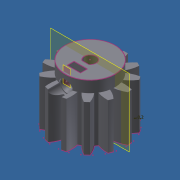
# Autodesk Inventor part: Stirnzahnrad2
Saved by Autodesk Inventor 2014 SP2 (Build 180246200, 246)
## iProperties
Created: 2014-12-12
Part Number: Stirnzahnrad2
Material: Steel
Document SubType Name: Modeling
Designer: 4ndreas
Categories: <?xml version="1.0" encoding="UTF-16"?> <MemberInstance><Categories><FamilyTemplate><FamilyTemplateParameter ValueType="xs:double" Id="1" ObjectReferenceKey="da_z" ObjectType="kUserParameterObject"/><FamilyTemplateParameter ValueType="xs:double" Id="2" ObjectReferenceKey="da_b" ObjectType="kUserParameterObject"/><FamilyTemplateParameter ValueType="xs:double" Id="3" ObjectReferenceKey="da_beta" ObjectType="kUserParameterObject"/><FamilyTemplateParameter ValueType="xs:double" Id="4" ObjectReferenceKey="da_da" ObjectType="kUserParameterObject"/><FamilyTemplateParameter ValueType="xs:double" Id="5" ObjectReferenceKey="da_aw" ObjectType="kUserParameterObject"/><FamilyTemplateParameter ValueType="xs:string" Id="6" ObjectReferenceKey="EAIAABAAAACIAQAAAAAAAIAAAAAAAAAA" ObjectType="83910656" SubObjectId="SurfaceGeometry"/></FamilyTemplate><ParamToTemplateMap><ParamToTemplate CategoryParameter="//CategoryParameter[@InternalName='046C89C9-8512-4d59-83FE-43B91F4F132A']" TemplateParameter="1"/><ParamToTemplate CategoryParameter="//CategoryParameter[@InternalName='2552DF32-E462-4b46-AEBF-C6C7768E72AC']" TemplateParameter="2"/><ParamToTemplate CategoryParameter="//CategoryParameter[@InternalName='C9EE641D-15FC-4fae-A226-E94C4372FDD7']" TemplateParameter="3"/><ParamToTemplate><ParamToTemplate CategoryParameter="//CategoryParameter[@InternalName='00B6519A-459B-49c7-AD84-2E56D39A5744']" ConstantValue="0.402671"/></ParamToTemplate><ParamToTemplate><ParamToTemplate CategoryParameter="//CategoryParameter[@InternalName='04B31F0E-C7A6-4894-AA32-9629BEFACF47']" ConstantValue="0.950000"/></ParamToTemplate><ParamToTemplate><ParamToTemplate CategoryParameter="//CategoryParameter[@InternalName='43CBEC2E-7847-49e7-A936-2F7889FCB2D9']" ConstantValue="0.500000"/></ParamToTemplate><ParamToTemplate><ParamToTemplate CategoryParameter="//CategoryParameter[@InternalName='B1EFC894-105D-4ebd-86BF-FA20ED196853']" ConstantValue="0.350000"/></ParamToTemplate><ParamToTemplate><ParamToTemplate CategoryParameter="//CategoryParameter[@InternalName='51175063-3D10-4879-93E8-6246FE8B403D']" ConstantValue="2060000000.000000"/></ParamToTemplate><ParamToTemplate><ParamToTemplate CategoryParameter="//CategoryParameter[@InternalName='A3A52E27-4454-46a9-B0BD-C932399B70AF']" ConstantValue="0.300000"/></ParamToTemplate><ParamToTemplate><ParamToTemplate CategoryParameter="//CategoryParameter[@InternalName='91B76062-C214-41d9-B1B9-14D2AB99603D']" ConstantValue="0.200000"/></ParamToTemplate><ParamToTemplate><ParamToTemplate CategoryParameter="//CategoryParameter[@InternalName='374E806E-8B8A-4dda-A9AA-1039D6500AD2']" ConstantValue="5.000000"/></ParamToTemplate><ParamToTemplate><ParamToTemplate CategoryParameter="//CategoryParameter[@InternalName='2D373A89-B862-43d6-8D0B-0CBF12AB9F6C']" ConstantValue="0.349066"/></ParamToTemplate><ParamToTemplate CategoryParameter="//CategoryParameter[@InternalName='37777632-D6A2-4fac-9D53-DB8ACD95C989']" TemplateParameter="4"/><ParamToTemplate CategoryParameter="//CategoryParameter[@InternalName='FD1017F1-B727-4f7e-9707-0F86F1FF9423']" TemplateParameter="5"/><ParamToTemplate><ParamToTemplate CategoryParameter="//CategoryParameter[@InternalName='9E1B4470-B2D3-4ff1-B813-535BB4CDF51A']" ConstantValue="3520000.000000"/></ParamToTemplate><ParamToTemplate><ParamToTemplate CategoryParameter="//CategoryParameter[@InternalName='F8452263-BFF6-458c-9FB1-07C4B99E95CD']" ConstantValue="11400000.000000"/></ParamToTemplate><ParamToTemplate><ParamToTemplate CategoryParameter="//CategoryParameter[@InternalName='3E3BB259-FD49-497f-8171-6EBC954A3479']" ConstantValue="2.000000"/></ParamToTemplate><ParamToTemplate CategoryParameter="//CategoryParameter[@InternalName='27C3BAF2-7550-4e4b-AE2C-0DB134B7D9B7']" TemplateParameter="6"/></ParamToTemplateMap><Category DisplayName="Gear" InternalName="DC85795E-93AB-48d5-8EEE-5A27447B64BD" Mnemonic="Gear"><CategoryParameter DisplayName="z" InternalName="046C89C9-8512-4d59-83FE-43B91F4F132A" Mnemonic="z"/><CategoryParameter DisplayName="b" InternalName="2552DF32-E462-4b46-AEBF-C6C7768E72AC" Mnemonic="b"/><CategoryParameter DisplayName="||b|" InternalName="C9EE641D-15FC-4fae-A226-E94C4372FDD7" Mnemonic="beta"/><CategoryParameter DisplayName="x" InternalName="00B6519A-459B-49c7-AD84-2E56D39A5744" Mnemonic="x"/><CategoryParameter DisplayName="a*" InternalName="04B31F0E-C7A6-4894-AA32-9629BEFACF47" Mnemonic="a"/><CategoryParameter DisplayName="c*" InternalName="43CBEC2E-7847-49e7-A936-2F7889FCB2D9" Mnemonic="c"/><CategoryParameter DisplayName="r|.f|*" InternalName="B1EFC894-105D-4ebd-86BF-FA20ED196853" Mnemonic="rf"/><CategoryParameter DisplayName="E" InternalName="51175063-3D10-4879-93E8-6246FE8B403D" Mnemonic="E"/><CategoryParameter DisplayName="||m|" InternalName="A3A52E27-4454-46a9-B0BD-C932399B70AF" Mnemonic="mi"/><Category DisplayName="SpurGear" InternalName="26C5A22E-A91E-4dfd-A3B3-23CCAFAE1764" Mnemonic="SpurGear"><CategoryParameter DisplayName="m" InternalName="91B76062-C214-41d9-B1B9-14D2AB99603D" Mnemonic="m"/><CategoryParameter DisplayName="P" InternalName="374E806E-8B8A-4dda-A9AA-1039D6500AD2" Mnemonic="PP"/><CategoryParameter DisplayName="||a|" InternalName="2D373A89-B862-43d6-8D0B-0CBF12AB9F6C" Mnemonic="alpha"/><CategoryParameter DisplayName="d|.a|" InternalName="37777632-D6A2-4fac-9D53-DB8ACD95C989" Mnemonic="da"/><CategoryParameter DisplayName="a|.w|" InternalName="FD1017F1-B727-4f7e-9707-0F86F1FF9423" Mnemonic="aw"/><CategoryParameter DisplayName="||s||.Flim|" InternalName="9E1B4470-B2D3-4ff1-B813-535BB4CDF51A" Mnemonic="sFlim"/><CategoryParameter DisplayName="||s||.Hlim|" InternalName="F8452263-BFF6-458c-9FB1-07C4B99E95CD" Mnemonic="sHlim"/><CategoryParameter DisplayName="Typ" InternalName="3E3BB259-FD49-497f-8171-6EBC954A3479" Mnemonic="type"/><CategoryParameter DisplayName="PitchDiameter" InternalName="27C3BAF2-7550-4e4b-AE2C-0DB134B7D9B7" Mnemonic="IDS_PITCHDIAM"/></Category></Category></Categories></MemberInstance>
Density: 1 g/cm^3
Appearance: Steel
CustomPartVersion: 1
Author: 4ndreas
Autodesk Inventor part; units mm, degrees
sketch "Sketch1" plane through (0, 0, 0) normal (0, 0, 1) x (1, 0, 0)
  circle A0 centre (0, 0) radius 15.6768
  dimension "d0" = 31.3535
  constraints: 1 centre point
  measures "d0" diameter of A0
extrude "Extrusion1" add sketch "Sketch1" along normal blind 20
ref_plane "Work Plane2" through (0, 0, 10) normal (0, 0, 1) x (1, 0, 0)
sketch "Sketch2" plane through (0, 0, 0) normal (0, 0, -1) x (-1, 0, 0)
  circle A0 centre (0, 0) radius 15.6768 projected
  circle A1 centre (0, 0) radius 13.1311
  dimension "d3" = 26.2623
  constraints: 1 centre point, 1 coincident
  measures "d3" diameter of A1
surface extrude "Flankendurchmesser" sketch "Sketch2" against normal through all shown no curves A1
ref_plane "Work Plane8" through (0, 0, 0) normal (0.9709418, 0.2393157, 0) x (0, 0, 1)
ref_plane "Work Plane9" through (0, 0, 0) normal (1, 0, 0) x (0, 1, 0)
spur gear teeth "Stirnzahnrad" teeth 13 pitch diameter 26 tip diameter 31.3535 root diameter 21.8107 face width 20 start plane through (0, 0, 0) normal (0, 0, -1) x (-1, 0, 0)
sketch "Skizze3" plane through (0, 0, 20) normal (0, 0, 1) x (1, 0, 0)
  arc A0 (-6.7255, 8.5845) -> (-7.7112, 7.7112) centre (0, 0) ccw projected
  arc A1 (-6.4339, 14.2956) -> (-8.1102, 13.4159) centre (0, 0) ccw projected
  circle A2 centre (0, 0) radius 10.9053
  constraints: 1 centre point, 1 coincident, 1 concentric
extrude "Extrusion2" add sketch "Skizze3" along normal blind 7
sketch "Skizze4" plane through (0, 0, 27) normal (0, 0, 1) x (1, 0, 0)
  circle A0 centre (0, 0) radius 10.9053 projected
  line L0 (-10.9053, 0) -> (10.9053, 0)
  constraints: 2 end point, 2 point on circle, 1 horizontal, 1 midpoint
ref_plane "Arbeitsebene11" through (-10.9053, 0, 27) normal (0, -1, 0) x (1, 0, 0)
hole "Bohrung1" at (0, 0, 27) direction (0, 0, -1) diameter 5.2 end through all
sketch "Skizze6" plane through (0, 0, 27) normal (0, 0, 1) x (1, 0, 0)
  circle A0 centre (0, 0) radius 2.6 projected
  circle A1 centre (0, 0) radius 10.9053 projected
  line L0 (-1.4913, -2.1298) -> (1.4913, -2.1298)
  line L1 (-1.4913, -2.1298) -> (-4.533, 0) construction
  line L2 (-4.533, 0) -> (0, 0) construction
  dimension "d63" = 35
  constraints: 6 end point, 2 point on circle, 1 horizontal, 1 parallel, 1 tangent
  measures "d63" angle of L1 L2
extrude "Extrusion4" add sketch "Skizze6" against normal up to surface (27 mm away) contours L0 A0 picked at (0.3106, -2.229)
sketch "Skizze5" plane through (-10.9053, 0, 27) normal (0, -1, 0) x (1, 0, 0)
  line L0 (10.2469, -27) -> (11.5638, -27) projected
  line L1 (-2.6508, -7) -> (0, -7) projected
  line L2 (0, -7) -> (0, 0) projected
  line L3 (13.5053, 0) -> (21.8107, 0) projected
  line L4 (21.8107, 0) -> (21.8107, -7) projected
  line L5 (21.8107, -7) -> (24.4615, -7) projected
  line L6 (24.4615, -7) -> (24.4615, -27) projected
  line L7 (24.4615, -27) -> (13.5053, -27) projected
  line L8 (-2.6508, -27) -> (-2.6508, -7) projected
  line L9 (0, -7) -> (21.8107, -7)
  circle A0 centre (10.9053, -7) radius 1.6
  line L10 (13.5053, -27) -> (13.5053, 0) projected
  line L11 (0, 0) -> (8.3053, 0) projected
  line L12 (8.3053, 0) -> (8.3053, -27) projected
  line L13 (8.3053, -27) -> (-2.6508, -27) projected
  point P0 (10.9053, -27)
  dimension "d52" = 3.2
  constraints: 2 end point, 1 centre point, 1 midpoint, 1 perpendicular
  measures "d52" diameter of A0
extrude "Extrusion3" cut sketch "Skizze5" along normal through all contours A0 L9 | L9 A0
sketch "Skizze7" plane through (0, 0, 27) normal (0, 0, 1) x (1, 0, 0)
  line L0 (1.4913, -2.1298) -> (-1.4913, -2.1298) projected
  circle A0 centre (0, 0) radius 10.9053 projected
  line L1 (-2.9, -4.1298) -> (2.9, -4.1298)
  line L2 (2.9, -4.1298) -> (2.9, -7.1298)
  line L3 (2.9, -7.1298) -> (-2.9, -7.1298)
  line L4 (-2.9, -7.1298) -> (-2.9, -4.1298)
  line L5 (0, 0) -> (0, -10.9053) construction
  dimension "d66" = 3
  dimension "d67" = 5.8
  dimension "d68" = 2
  constraints: 10 end point, 3 parallel, 1 horizontal, 1 perpendicular, 1 vertical alignment, 2 other
  measures "d66" distance between parallel lines of L3 L1
  measures "d67" distance between parallel lines of L2 L4
  measures "d68" distance between parallel lines of L1 L0
extrude "Extrusion5" cut sketch "Skizze7" against normal blind 12 contours L1 L2 L3 L4
ref_plane "Arbeitsebene12" through (-1.4913, -10.1298, 27) normal (0, 1, 0) x (1, 0, 0)
sketch "Skizze8" plane through (-1.4913, -10.1298, 27) normal (0, 1, 0) x (1, 0, 0)
  circle A0 centre (1.4913, 7) radius 1.6 projected
  line L0 (-2.5477, 0) -> (-2.5477, 7) projected
  line L1 (-2.5477, 7) -> (-3.0246, 7) projected
  line L2 (-3.0246, 7) -> (-3.0246, 27) projected
  line L3 (-3.0246, 27) -> (6.0072, 27) projected
  line L4 (6.0072, 27) -> (6.0072, 7) projected
  line L5 (6.0072, 7) -> (5.5303, 7) projected
  line L6 (5.5303, 7) -> (5.5303, 0) projected
  line L7 (5.5303, 0) -> (-2.5477, 0) projected
  line L8 (12.2006, 7) -> (7.9327, 7) projected
  line L9 (7.9327, 7) -> (7.9327, 27) projected
  line L10 (7.9327, 27) -> (12.2006, 27) projected
  line L11 (12.2006, 27) -> (12.2006, 7) projected
  line L12 (-4.9502, 7) -> (-9.218, 7) projected
  line L13 (-9.218, 7) -> (-9.218, 27) projected
  line L14 (-9.218, 27) -> (-4.9502, 27) projected
  line L15 (-4.9502, 27) -> (-4.9502, 7) projected
  circle A1 centre (1.4913, 7) radius 3
  point P0 (1.4913, 27)
  dimension "d72" = 6
  constraints: 1 centre point, 1 coincident
  measures "d72" diameter of A1
extrude "Extrusion6" cut sketch "Skizze8" against normal blind 12 contours A1
chamfer "Fase1" distance 1 angle 45 1 edges at (-1.6, -10.1298, 20)
sketch "Skizze10" plane through (0, 0, 27) normal (0, 0, 1) x (1, 0, 0)
  line L0 (-2.9, -7.1298) -> (-2.9, -4.1298) projected
  line L1 (-2.9, -4.1298) -> (2.9, -4.1298) projected
  line L2 (2.9, -4.1298) -> (2.9, -7.1298) projected
  line L3 (2.9, -7.1298) -> (-2.9, -7.1298) projected
  arc A0 (1.4913, -2.1298) -> (-1.4913, -2.1298) centre (0, 0) ccw projected
  line L4 (1.4913, -2.1298) -> (-1.4913, -2.1298) projected
  circle A1 centre (0, 0) radius 10.9053 projected
extrude "Extrusion7" cut sketch "Skizze10" against normal blind 2
sketch "Skizze11" plane through (0, 0, 0) normal (0, 0, -1) x (-1, 0, 0)
  arc A0 (1.4913, -2.1298) -> (-1.4913, -2.1298) centre (0, 0) ccw projected
  line L0 (-1.4913, -2.1298) -> (1.4913, -2.1298) projected
  arc A1 (6.7255, 8.5845) -> (8.1102, 13.4159) centre (-5.623, 14.7376) ccw projected
  arc A2 (8.1102, 13.4159) -> (6.4339, 14.2956) centre (0, 0) ccw projected
  arc A3 (6.4339, 14.2956) -> (3.2444, 10.4116) centre (15.323, 3.7443) ccw projected
  arc A4 (3.2444, 10.4116) -> (1.9657, 10.7267) centre (0, 0) ccw projected
  arc A5 (1.9657, 10.7267) -> (0.9465, 15.6482) centre (-11.8278, 10.4364) ccw projected
  arc A6 (0.9465, 15.6482) -> (-0.9465, 15.6482) centre (0, 0) ccw projected
  arc A7 (-0.9465, 15.6482) -> (-1.9657, 10.7267) centre (11.8278, 10.4364) ccw projected
  arc A8 (-1.9657, 10.7267) -> (-3.2444, 10.4116) centre (0, 0) ccw projected
  arc A9 (-3.2444, 10.4116) -> (-6.4339, 14.2956) centre (-15.323, 3.7443) ccw projected
  arc A10 (-6.4339, 14.2956) -> (-8.1102, 13.4159) centre (0, 0) ccw projected
  arc A11 (-8.1102, 13.4159) -> (-6.7255, 8.5845) centre (5.623, 14.7376) ccw projected
  arc A12 (-6.7255, 8.5845) -> (-7.7112, 7.7112) centre (0, 0) ccw projected
  arc A13 (-7.7112, 7.7112) -> (-12.3405, 9.6682) centre (-15.308, -3.8056) ccw projected
  arc A14 (-12.3405, 9.6682) -> (-13.4159, 8.1102) centre (0, 0) ccw projected
  arc A15 (-13.4159, 8.1102) -> (-9.9446, 4.4757) centre (-1.87, 15.6627) ccw projected
  arc A16 (-9.9446, 4.4757) -> (-10.4116, 3.2444) centre (0, 0) ccw projected
  arc A17 (-10.4116, 3.2444) -> (-15.42, 2.8258) centre (-11.786, -10.4836) ccw projected
  arc A18 (-15.42, 2.8258) -> (-15.6482, 0.9465) centre (0, 0) ccw projected
  arc A19 (-15.6482, 0.9465) -> (-10.8854, -0.6584) centre (-8.9346, 12.9995) ccw projected
  arc A20 (-10.8854, -0.6584) -> (-10.7267, -1.9657) centre (0, 0) ccw projected
  arc A21 (-10.7267, -1.9657) -> (-14.9669, -4.6639) centre (-5.564, -14.76) ccw projected
  arc A22 (-14.9669, -4.6639) -> (-14.2956, -6.4339) centre (0, 0) ccw projected
  arc A23 (-14.2956, -6.4339) -> (-9.3326, -5.6417) centre (-13.9524, 7.3584) ccw projected
  arc A24 (-9.3326, -5.6417) -> (-8.5845, -6.7255) centre (0, 0) ccw projected
  arc A25 (-8.5845, -6.7255) -> (-11.0851, -11.0851) centre (1.9326, -15.6551) ccw projected
  arc A26 (-11.0851, -11.0851) -> (-9.6682, -12.3405) centre (0, 0) ccw projected
  arc A27 (-9.6682, -12.3405) -> (-5.6417, -9.3326) centre (-15.7739, 0.0315) ccw projected
  arc A28 (-5.6417, -9.3326) -> (-4.4757, -9.9446) centre (0, 0) ccw projected
  arc A29 (-4.4757, -9.9446) -> (-4.6639, -14.9669) centre (8.9865, -12.9637) ccw projected
  arc A30 (-4.6639, -14.9669) -> (-2.8258, -15.42) centre (0, 0) ccw projected
  arc A31 (-2.8258, -15.42) -> (-0.6584, -10.8854) centre (-13.9817, -7.3026) ccw projected
  arc A32 (-0.6584, -10.8854) -> (0.6584, -10.8854) centre (0, 0) ccw projected
  arc A33 (0.6584, -10.8854) -> (2.8258, -15.42) centre (13.9817, -7.3026) ccw projected
  arc A34 (2.8258, -15.42) -> (4.6639, -14.9669) centre (0, 0) ccw projected
  arc A35 (4.6639, -14.9669) -> (4.4757, -9.9446) centre (-8.9865, -12.9637) ccw projected
  arc A36 (4.4757, -9.9446) -> (5.6417, -9.3326) centre (0, 0) ccw projected
  arc A37 (5.6417, -9.3326) -> (9.6682, -12.3405) centre (15.7739, 0.0315) ccw projected
  arc A38 (9.6682, -12.3405) -> (11.0851, -11.0851) centre (0, 0) ccw projected
  arc A39 (11.0851, -11.0851) -> (8.5845, -6.7255) centre (-1.9326, -15.6551) ccw projected
  arc A40 (8.5845, -6.7255) -> (9.3326, -5.6417) centre (0, 0) ccw projected
  arc A41 (9.3326, -5.6417) -> (14.2956, -6.4339) centre (13.9524, 7.3584) ccw projected
  arc A42 (14.2956, -6.4339) -> (14.9669, -4.6639) centre (0, 0) ccw projected
  arc A43 (14.9669, -4.6639) -> (10.7267, -1.9657) centre (5.564, -14.76) ccw projected
  arc A44 (10.7267, -1.9657) -> (10.8854, -0.6584) centre (0, 0) ccw projected
  arc A45 (10.8854, -0.6584) -> (15.6482, 0.9465) centre (8.9346, 12.9995) ccw projected
  arc A46 (15.6482, 0.9465) -> (15.42, 2.8258) centre (0, 0) ccw projected
  arc A47 (15.42, 2.8258) -> (10.4116, 3.2444) centre (11.786, -10.4836) ccw projected
  arc A48 (10.4116, 3.2444) -> (9.9446, 4.4757) centre (0, 0) ccw projected
  arc A49 (9.9446, 4.4757) -> (13.4159, 8.1102) centre (1.87, 15.6627) ccw projected
  arc A50 (13.4159, 8.1102) -> (12.3405, 9.6682) centre (0, 0) ccw projected
  arc A51 (12.3405, 9.6682) -> (7.7112, 7.7112) centre (15.308, -3.8056) ccw projected
  arc A52 (7.7112, 7.7112) -> (6.7255, 8.5845) centre (0, 0) ccw projected
  arc A53 (-6.4667, 14.061) -> (-7.8984, 13.3096) centre (0, 0) ccw
  arc A54 (-3.341, 10.1707) -> (-6.4667, 14.061) centre (-15.323, 3.7443) ccw
  arc A55 (-1.7683, 10.5583) -> (-3.341, 10.1707) centre (0, 0) ccw
  arc A56 (-0.8085, 15.4556) -> (-1.7683, 10.5583) centre (11.8278, 10.4364) ccw
  arc A57 (0.8085, 15.4556) -> (-0.8085, 15.4556) centre (0, 0) ccw
  arc A58 (1.7683, 10.5583) -> (0.8085, 15.4556) centre (-11.8278, 10.4364) ccw
  arc A59 (3.341, 10.1707) -> (1.7683, 10.5583) centre (0, 0) ccw
  arc A60 (6.4667, 14.061) -> (3.341, 10.1707) centre (15.323, 3.7443) ccw
  arc A61 (7.8984, 13.3096) -> (6.4667, 14.061) centre (0, 0) ccw
  arc A62 (6.4724, 8.5272) -> (7.8984, 13.3096) centre (-5.623, 14.7376) ccw
  arc A63 (7.6848, 7.453) -> (6.4724, 8.5272) centre (0, 0) ccw
  arc A64 (12.2605, 9.4451) -> (7.6848, 7.453) centre (15.308, -3.8056) ccw
  arc A65 (13.179, 8.1145) -> (12.2605, 9.4451) centre (0, 0) ccw
  arc A66 (9.6938, 4.5426) -> (13.179, 8.1145) centre (1.87, 15.6627) ccw
  arc A67 (10.2682, 3.028) -> (9.6938, 4.5426) centre (0, 0) ccw
  arc A68 (15.2455, 2.6655) -> (10.2682, 3.028) centre (11.786, -10.4836) ccw
  arc A69 (15.4404, 1.0604) -> (15.2455, 2.6655) centre (0, 0) ccw
  arc A70 (10.6945, -0.4827) -> (15.4404, 1.0604) centre (8.9346, 12.9995) ccw
  arc A71 (10.4992, -2.0907) -> (10.6945, -0.4827) centre (0, 0) ccw
  arc A72 (14.7379, -4.7247) -> (10.4992, -2.0907) centre (5.564, -14.76) ccw
  arc A73 (14.1646, -6.2366) -> (14.7379, -4.7247) centre (0, 0) ccw
  arc A74 (9.2451, -5.3974) -> (14.1646, -6.2366) centre (13.9524, 7.3584) ccw
  arc A75 (8.325, -6.7304) -> (9.2451, -5.3974) centre (0, 0) ccw
  arc A76 (10.8541, -11.0326) -> (8.325, -6.7304) centre (-1.9326, -15.6551) ccw
  arc A77 (9.6438, -12.1048) -> (10.8541, -11.0326) centre (0, 0) ccw
  arc A78 (5.6779, -9.0756) -> (9.6438, -12.1048) centre (15.7739, 0.0315) ccw
  arc A79 (4.2436, -9.8283) -> (5.6779, -9.0756) centre (0, 0) ccw
  arc A80 (4.4837, -14.813) -> (4.2436, -9.8283) centre (-8.9865, -12.9637) ccw
  arc A81 (2.9138, -15.2) -> (4.4837, -14.813) centre (0, 0) ccw
  arc A82 (0.8099, -10.6747) -> (2.9138, -15.2) centre (13.9817, -7.3026) ccw
  arc A83 (-0.8099, -10.6747) -> (0.8099, -10.6747) centre (0, 0) ccw
  arc A84 (-2.9138, -15.2) -> (-0.8099, -10.6747) centre (-13.9817, -7.3026) ccw
  arc A85 (-4.4837, -14.813) -> (-2.9138, -15.2) centre (0, 0) ccw
  arc A86 (-4.2436, -9.8283) -> (-4.4837, -14.813) centre (8.9865, -12.9637) ccw
  arc A87 (-5.6779, -9.0756) -> (-4.2436, -9.8283) centre (0, 0) ccw
  arc A88 (-9.6438, -12.1048) -> (-5.6779, -9.0756) centre (-15.7739, 0.0315) ccw
  arc A89 (-10.8541, -11.0326) -> (-9.6438, -12.1048) centre (0, 0) ccw
  arc A90 (-8.325, -6.7304) -> (-10.8541, -11.0326) centre (1.9326, -15.6551) ccw
  arc A91 (-9.2451, -5.3974) -> (-8.325, -6.7304) centre (0, 0) ccw
  arc A92 (-14.1646, -6.2366) -> (-9.2451, -5.3974) centre (-13.9524, 7.3584) ccw
  arc A93 (-14.7379, -4.7247) -> (-14.1646, -6.2366) centre (0, 0) ccw
  arc A94 (-10.4992, -2.0907) -> (-14.7379, -4.7247) centre (-5.564, -14.76) ccw
  arc A95 (-10.6945, -0.4827) -> (-10.4992, -2.0907) centre (0, 0) ccw
  arc A96 (-15.4404, 1.0604) -> (-10.6945, -0.4827) centre (-8.9346, 12.9995) ccw
  arc A97 (-15.2455, 2.6655) -> (-15.4404, 1.0604) centre (0, 0) ccw
  arc A98 (-10.2682, 3.028) -> (-15.2455, 2.6655) centre (-11.786, -10.4836) ccw
  arc A99 (-9.6938, 4.5426) -> (-10.2682, 3.028) centre (0, 0) ccw
  arc A100 (-13.179, 8.1145) -> (-9.6938, 4.5426) centre (-1.87, 15.6627) ccw
  arc A101 (-12.2605, 9.4451) -> (-13.179, 8.1145) centre (0, 0) ccw
  arc A102 (-7.6848, 7.453) -> (-12.2605, 9.4451) centre (-15.308, -3.8056) ccw
  arc A103 (-6.4724, 8.5272) -> (-7.6848, 7.453) centre (0, 0) ccw
  arc A104 (-7.8984, 13.3096) -> (-6.4724, 8.5272) centre (5.623, 14.7376) ccw
  dimension "d80" = 0.2
  constraints: 104 point on circle, 52 centre point, 51 other
  measures "d80" radial gap between concentric circles of A53 A10
sketch "Skizze12" plane through (0, 0, 25) normal (0, 0, 1) x (1, 0, 0)
  line L0 (-1.4913, -2.1298) -> (1.4913, -2.1298) projected
  arc A0 (1.4913, -2.1298) -> (-1.4913, -2.1298) centre (0, 0) ccw projected
  line L1 (-2.9, -7.1298) -> (2.9, -7.1298) projected
  line L2 (-2.9, -4.1298) -> (-2.9, -7.1298) projected
  line L3 (2.9, -4.1298) -> (-2.9, -4.1298) projected
  line L4 (2.9, -7.1298) -> (2.9, -4.1298) projected
  circle A1 centre (0, 0) radius 10.9053 projected
equation "\"d0\" = da_da"
equation "\"d1\" = da_b"
equation "\"d3\" = da_dw"
equation "\"d16\" = da_aw"
equation "\"d43\" = da_aw"
equation "\"d46\" = da_aw"
equation "\"da_da\" = 31.353516"
equation "\"da_b\" = 20"
equation "\"da_dw\" = 26.262282"
equation "\"da_aw\" = 77.776758"
body "Solid1"
body "Srf1"
